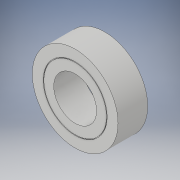
# Autodesk Inventor part: RobotArm ShaftColar
Saved by Autodesk Inventor 2018 (Build 220112000, 112)
## iProperties
Created: 2018-01-20
Part Number: RobotArm ShaftColar
Material: Generic
Document SubType Name: Modeling
Designer: lopez.xavier
Density: 1 g/cm^3
Appearance: Default
Author: lopez.xavier
Autodesk Inventor part; units mm, degrees
ref_plane "YZ Plane" through (0, 0, 0) normal (1, 0, 0) x (0, 1, 0)
ref_plane "XZ Plane" through (0, 0, 0) normal (0, 1, 0) x (-1, 0, 0)
ref_plane "XY Plane" through (0, 0, 0) normal (0, 0, 1) x (1, 0, 0)
sketch "Sketch1" plane through (0, 0, 0) normal (0, 0, 1) x (1, 0, 0)
  circle A0 centre (0, 0) radius 16.51
  circle A1 centre (0, 0) radius 8.255
  dimension "d0" = 33.02
  dimension "d3" = 16.51
  constraints: 2 centre point, 2 coincident
  measures "d0" diameter of A0
  measures "d3" diameter of A1
extrude "Extrusion2" add sketch "Sketch1" along normal blind 11.43
sketch "Sketch2" plane through (0, 0, 11.43) normal (0, 0, 1) x (1, 0, 0)
  circle A0 centre (0, 0) radius 12.065
  circle A1 centre (0, 0) radius 12.319
  circle A2 centre (0, 0) radius 8.255 projected
  dimension "d6" = 0.254
  dimension "d8" = 3.81
  constraints: 2 centre point, 2 coincident
  measures "d6" radial gap between concentric circles of A1 A0
  measures "d8" radial gap between concentric circles of A2 A0
extrude "Extrusion3" cut sketch "Sketch2" against normal blind 0.254 contours A1
body "Solid2"
